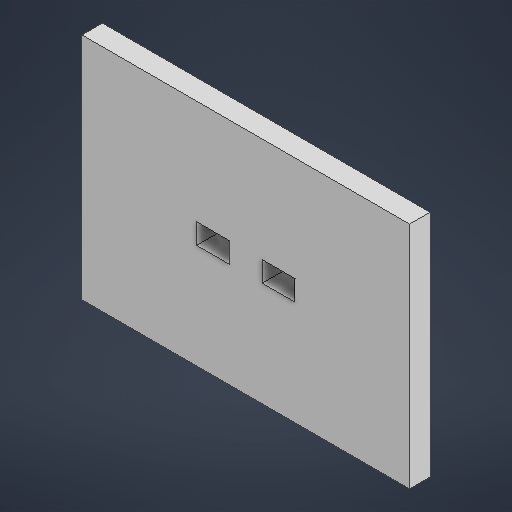
# Autodesk Inventor part: pitahaya4
Saved by Autodesk Inventor 2026.3 (Build 303398000, 398)
## iProperties
Created: 2026-09-15
Part Number: pitahaya4
Material: Generic
Document SubType Name: Modeling
Designer: micha
Density: 1 g/cm^3
Appearance: Default
Author: micha
Autodesk Inventor part; units mm, degrees
ref_plane "YZ Plane" through (0, 0, 0) normal (1, 0, 0) x (0, 1, 0)
ref_plane "XZ Plane" through (0, 0, 0) normal (0, 1, 0) x (-1, 0, 0)
ref_plane "XY Plane" through (0, 0, 0) normal (0, 0, 1) x (1, 0, 0)
sketch "Sketch1" plane through (0, 0, 0) normal (0, 0, 1) x (1, 0, 0)
  line L0 (0, 8.7149) -> (0, -8.7149) construction
  line L1 (-12.4402, 0) -> (12.4402, 0) construction
  line L2 (-20, 14) -> (20, 14)
  line L3 (20, 14) -> (20, -14)
  line L4 (20, -14) -> (-20, -14)
  line L5 (-20, -14) -> (-20, 14)
  line L6 (-6, 1.25) -> (-2, 1.25)
  line L7 (-2, 1.25) -> (-2, -1.25)
  line L8 (-2, -1.25) -> (-6, -1.25)
  line L9 (-6, -1.25) -> (-6, 1.25)
  line L10 (2, 1.25) -> (6, 1.25)
  line L11 (6, 1.25) -> (6, -1.25)
  line L12 (6, -1.25) -> (2, -1.25)
  line L13 (2, -1.25) -> (2, 1.25)
  point P0 (0, 0)
  point P1 (0, 0)
  dimension "d0" = 4
  dimension "d1" = 4
  dimension "d2" = 4
  dimension "d3" = 2.5
  dimension "d4" = 28
  dimension "d5" = 40
  constraints: 28 end point, 6 parallel, 4 horizontal, 3 perpendicular, 2 horizontal alignment, 2 midpoint, 1 coincident, 1 vertical, 4 other
  measures "d0" distance of L6.start L6.end
  measures "d1" distance of L10.start L10.end
  measures "d2" distance between parallel lines of L13 L7
  measures "d3" distance of L8.end L6.start
  measures "d4" distance of L4.end L2.start
  measures "d5" distance of L3.end L4.end
extrude "Extrusion1" add sketch "Sketch1" along normal mid plane 2.5
body "Solid1"
